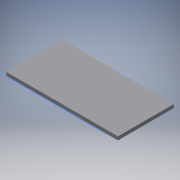
# Autodesk Inventor part: base
Saved by Autodesk Inventor 2016 (Build 200138000, 138)
## iProperties
Created: 2016-01-27
Part Number: base
Material: Generic
Document SubType Name: Modeling
Designer: seve
Density: 1 g/cm^3
Appearance: Default
Author: seve
Autodesk Inventor part; units mm, degrees
ref_plane "YZ Plane" through (0, 0, 0) normal (1, 0, 0) x (0, 1, 0)
ref_plane "XZ Plane" through (0, 0, 0) normal (0, 1, 0) x (-1, 0, 0)
ref_plane "XY Plane" through (0, 0, 0) normal (0, 0, 1) x (1, 0, 0)
sketch "Sketch1" plane through (0, 0, 0) normal (0, 1, 0) x (-1, 0, 0)
  line L0 (-3.4011, 4.0367) -> (72.7989, 4.0367)
  line L1 (72.7989, 4.0367) -> (72.7989, -21.3633)
  line L2 (72.7989, -21.3633) -> (-3.4011, -21.3633)
  line L3 (-3.4011, -21.3633) -> (-3.4011, 4.0367)
  point P0 (0, 0)
  dimension "d0" = 76.2
  dimension "d1" = 25.4
  constraints: 8 end point, 2 parallel, 1 horizontal, 1 perpendicular
  measures "d0" distance of L1.end L2.end
  measures "d1" distance of L0.end L1.end
extrude "Extrusion1" add sketch "Sketch1" along normal blind 3.175
body "Solid1"
